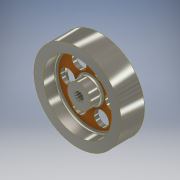
# Autodesk Inventor part: reverse gear fly wheel
Saved by Autodesk Inventor 2017 (Build 210142000, 142)
## iProperties
Created: 2018-11-09
Part Number: reverse gear fly wheel
Material: Generic
Document SubType Name: Modeling
Designer: User
Density: 1 g/cm^3
Appearance: Default
Author: User
Autodesk Inventor part; units mm, degrees
ref_plane "XY Plane" through (0, 0, 0) normal (0, 0, 1) x (1, 0, 0)
sketch "Sketch1" plane through (0, 0, 0) normal (0, 1, 0) x (-1, 0, 0)
  circle A0 centre (0, 0) radius 41
  dimension "d0" = 82
  constraints: 1 centre point, 1 coincident
  measures "d0" diameter of A0
extrude "Extrusion1" add sketch "Sketch1" along normal blind 22
sketch "Sketch2" plane through (0, 22, 0) normal (0, 1, 0) x (1, 0, 0)
  circle A0 centre (0, 0) radius 32
  dimension "d3" = 64
  constraints: 1 centre point, 1 coincident
  measures "d3" diameter of A0
extrude "Extrusion2" cut sketch "Sketch2" against normal blind 6
sketch "Sketch3" plane through (0, 0, 0) normal (0, -1, 0) x (1, 0, 0)
  circle A0 centre (0, 0) radius 32
  dimension "d6" = 64
  constraints: 1 centre point, 1 coincident
  measures "d6" diameter of A0
extrude "Extrusion3" cut sketch "Sketch3" against normal blind 12
ref_plane "Work Plane1" through (0, 1.5, 0) normal (0, 1, 0) x (-1, 0, 0)
sketch "Sketch4" plane through (0, 1.5, 0) normal (0, 1, 0) x (-1, 0, 0)
  circle A0 centre (0, 0) radius 11
  dimension "d10" = 22
  constraints: 1 centre point, 1 coincident
  measures "d10" diameter of A0
extrude "Extrusion4" add sketch "Sketch4" along normal blind 22
sketch "Sketch5" plane through (0, 23.5, 0) normal (0, 1, 0) x (1, 0, 0)
  circle A0 centre (0, 0) radius 4
  dimension "d13" = 8
  constraints: 1 centre point, 1 coincident
  measures "d13" diameter of A0
extrude "Extrusion5" cut sketch "Sketch5" against normal through all
ref_plane "Work Plane2" through (-11, 0, 0) normal (1, 0, 0) x (0, 1, 0)
sketch "Sketch6" plane through (-11, 0, 0) normal (1, 0, 0) x (0, 1, 0)
  circle A0 centre (5.9844, 0) radius 1.5
  point P0 (0, 0)
  dimension "d17" = 3
  dimension "d33" = 5.9844
  constraints: 1 centre point
  measures "d17" diameter of A0
  measures "d33" distance of point (0, 0) A0.centre
extrude "Extrusion6" cut sketch "Sketch6" along normal blind 10
sketch "Sketch7" plane through (0, 12, 0) normal (0, -1, 0) x (1, 0, 0)
  circle A0 centre (20.9744, 0) radius 7
  circle A1 centre (10.4872, 18.1643) radius 7
  circle A2 centre (-10.4872, 18.1643) radius 7
  circle A3 centre (-20.9744, 0) radius 7
  circle A4 centre (-10.4872, -18.1643) radius 7
  circle A5 centre (10.4872, -18.1643) radius 7
  point P0 (0, 0)
  dimension "d20" = 14
  dimension "d23" = 360
  dimension "d34" = 20.9744
  constraints: 6 centre point, 13 other
  measures "d20" diameter of A0
  measures "d34" distance of A0.centre point (0, 0)
extrude "Extrusion7" cut sketch "Sketch7" against normal through all
fillet "Fillet1" radius 2 1 edges at (11, 12, 0)
fillet "Fillet2" radius 2 1 edges at (-32, 12, 0)
fillet "Fillet3" radius 2 1 edges at (-32, 16, 0)
chamfer "Chamfer1" distance 1.6 angle 45 1 edges at (11, 23.5, 0)
body "Solid1"
